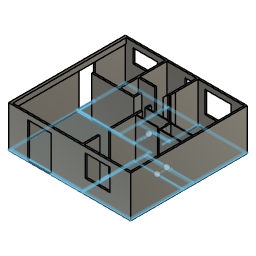
main (Autodesk Fusion 360 design; units mm, degrees)
Autodesk Fusion 360 part; units mm, degrees
note: some values were not read from the file. Set by a fixed rule: which sketch regions a step uses.
sketch "Sketch1" plane through (0, 0, 0) normal (0, 0, 1) x (1, 0, 0)
  line L0 (-340.048, 12.5122) -> (96.952, 12.5122)
  line L1 (96.952, 12.5122) -> (96.952, -391.4878)
  line L2 (96.952, -391.4878) -> (-340.048, -391.4878)
  line L3 (-340.048, -391.4878) -> (-340.048, 12.5122)
  line L4 (-350.048, 22.5122) -> (106.952, 22.5122)
  line L5 (106.952, 22.5122) -> (106.952, -401.4878)
  line L6 (106.952, -401.4878) -> (-350.048, -401.4878)
  line L7 (-350.048, -401.4878) -> (-350.048, 22.5122)
  line L8 (96.952, -391.4878) -> (106.952, -391.4878)
  line L9 (106.952, -391.4878) -> (392.952, -391.4878)
  line L10 (392.952, -391.4878) -> (392.952, -75.4878)
  line L11 (392.952, -75.4878) -> (106.952, -75.4878)
  line L12 (106.952, -75.4878) -> (106.952, -391.4878)
  line L13 (106.952, -401.4878) -> (402.952, -401.4878)
  line L14 (402.952, -401.4878) -> (402.952, -75.4878)
  line L15 (-340.048, 12.5122) -> (-340.048, 22.5122)
  line L16 (96.952, 12.5122) -> (96.952, 22.5122)
  line L17 (-340.048, 22.5122) -> (-93.048, 22.5122)
  line L18 (-93.048, 22.5122) -> (-93.048, 308.5122)
  line L19 (-93.048, 308.5122) -> (-340.048, 308.5122)
  line L20 (-340.048, 308.5122) -> (-340.048, 22.5122)
  line L21 (-350.048, 22.5122) -> (-83.048, 22.5122)
  line L22 (-83.048, 22.5122) -> (-83.048, 318.5122)
  line L23 (-83.048, 318.5122) -> (-350.048, 318.5122)
  line L24 (-350.048, 318.5122) -> (-350.048, 22.5122)
  line L25 (-93.048, 308.5122) -> (-83.048, 308.5122)
  line L26 (-83.048, 308.5122) -> (98.952, 308.5122)
  line L27 (98.952, 308.5122) -> (98.952, 141.5122)
  line L28 (98.952, 141.5122) -> (-83.048, 141.5122)
  line L29 (-83.048, 141.5122) -> (-83.048, 308.5122)
  line L30 (-83.048, 318.5122) -> (108.952, 318.5122)
  line L31 (108.952, 318.5122) -> (108.952, 131.5122)
  line L32 (-83.048, 131.5122) -> (108.952, 131.5122)
  line L33 (98.952, 308.5122) -> (108.952, 308.5122)
  line L34 (108.952, 308.5122) -> (392.952, 308.5122)
  line L35 (392.952, 308.5122) -> (392.952, -7.4878)
  line L36 (392.952, -7.4878) -> (106.952, -7.4878)
  line L37 (108.952, 318.5122) -> (402.952, 318.5122)
  line L38 (402.952, 318.5122) -> (402.952, -75.4878)
  line L39 (392.952, -75.4878) -> (402.952, -75.4878)
  line L40 (106.952, -7.4878) -> (232.2735, -7.4878)
  line L41 (249.952, -75.4878) -> (106.952, -75.4878)
  line L42 (106.952, -75.4878) -> (106.952, -7.4878)
  line L43 (240, -7.4878) -> (392.952, -7.4878)
  line L44 (392.952, -7.4878) -> (392.952, -75.4878)
  line L45 (392.952, -75.4878) -> (240, -75.4878)
  line L46 (106.952, -2.4878) -> (256.952, -2.4878)
  line L47 (256.952, -2.4878) -> (256.952, -20)
  line L48 (256.952, -20) -> (106.952, -20)
  line L49 (106.952, -20) -> (106.952, -2.4878)
  line L50 (392.952, -80.4878) -> (242.952, -80.4878)
  line L51 (242.952, -80.4878) -> (242.952, -20)
  line L52 (242.952, -20) -> (392.952, -20)
  line L53 (392.952, -20) -> (392.952, -80.4878)
  line L54 (106.952, -75.4878) -> (96.952, -75.4878)
  line L55 (96.952, -75.4878) -> (96.952, -230.4878)
  line L56 (96.952, -230.4878) -> (106.952, -230.4878)
  line L57 (106.952, -230.4878) -> (106.952, -75.4878)
  line L58 (96.952, -391.4878) -> (106.952, -391.4878)
  line L59 (106.952, -391.4878) -> (106.952, -295.4878)
  line L60 (106.952, -295.4878) -> (96.952, -295.4878)
  line L61 (96.952, -295.4878) -> (96.952, -391.4878)
  line L62 (-87.7265, -391.4878) -> (79.2735, -391.4878)
  line L63 (79.2735, -391.4878) -> (79.2735, -401.4878)
  line L64 (79.2735, -401.4878) -> (-87.7265, -401.4878)
  line L65 (-87.7265, -401.4878) -> (-87.7265, -391.4878)
  line L66 (-340.048, -391.4878) -> (-232.048, -391.4878)
  line L67 (-232.048, -391.4878) -> (-232.048, -401.4878)
  line L68 (-232.048, -401.4878) -> (-340.048, -401.4878)
  line L69 (-340.048, -401.4878) -> (-340.048, -391.4878)
  line L70 (-251.548, 22.5122) -> (8.452, 22.5122)
  line L71 (8.452, 22.5122) -> (8.452, 12.5122)
  line L72 (8.452, 12.5122) -> (-251.548, 12.5122)
  line L73 (-251.548, 12.5122) -> (-251.548, 22.5122)
  line L74 (-350.048, 22.5122) -> (-340.048, 22.5122)
  line L75 (-340.048, 22.5122) -> (-340.048, 122.5122)
  line L76 (-340.048, 122.5122) -> (-350.048, 122.5122)
  line L77 (-350.048, 122.5122) -> (-350.048, 22.5122)
  line L78 (8.452, 22.5122) -> (-1.548, 22.5122)
  line L79 (-1.548, 22.5122) -> (-1.548, 131.5122)
  line L80 (-1.548, 131.5122) -> (8.452, 131.5122)
  line L81 (8.452, 131.5122) -> (8.452, 22.5122)
  line L82 (-1.548, 131.5122) -> (8.452, 131.5122)
  line L83 (8.452, 131.5122) -> (8.452, 77.0122)
  line L84 (-1.548, 114.5) -> (-1.548, 131.5122)
  line L85 (-1.548, 61.5122) -> (8.452, 61.5122)
  line L86 (98.952, 141.5122) -> (99.322, 141.5122)
  line L87 (99.322, 141.5122) -> (99.322, 102.5122)
  line L88 (99.322, 102.5122) -> (98.952, 102.5122)
  line L89 (98.952, 102.5122) -> (98.952, 141.5122)
  line L90 (18.952, 141.5122) -> (98.952, 141.5122)
  line L91 (98.952, 141.5122) -> (98.952, 131.5122)
  line L92 (98.952, 131.5122) -> (18.952, 131.5122)
  line L93 (18.952, 131.5122) -> (18.952, 141.5122)
  dimension "d1" = 437
  dimension "d2" = 404
  dimension "d3" = 10
  dimension "d4" = 10
  dimension "d5" = 10
  dimension "d6" = 10
  dimension "d7" = 286
  dimension "d9" = 10
  dimension "d10" = 247
  dimension "d11" = 286
  dimension "d12" = 10
  dimension "d13" = 10
  dimension "d14" = 182
  dimension "d15" = 167
  dimension "d16" = 10
  dimension "d17" = 10
  dimension "d19" = 316
  dimension "d20" = 10
  dimension "d21" = 10
  dimension "d22" = 10
  dimension "d23" = 150
  dimension "d24" = 150
  dimension "d25" = 5
  dimension "d26" = 5
  dimension "d27" = 155
  dimension "d28" = 96
  dimension "d29" = 167
  dimension "d30" = 108
  dimension "d31" = 260
  dimension "d32" = 88.5
  dimension "d33" = 88.5
  dimension "d34" = 100
  dimension "d35" = 10
  dimension "d36" = 70
  dimension "d37" = 80
  dimension "d38" = 80
  dimension "d52" = 316
  constraint horizontal L0
  constraint vertical L1
  constraint horizontal L2
  constraint vertical L3
  constraint horizontal L4
  constraint vertical L5
  constraint horizontal L6
  constraint vertical L7
  constraint coincident L5 L8.end
  constraint perpendicular L5 L8
  constraint horizontal L9
  constraint vertical L10
  constraint horizontal L11
  constraint vertical L12
  constraint perpendicular L5 L13
  constraint perpendicular L13 L14
  constraint coincident L4 L15.end
  constraint perpendicular L4 L15
  constraint coincident L4 L16.end
  constraint perpendicular L4 L16
  constraint horizontal L17
  constraint vertical L18
  constraint horizontal L19
  constraint vertical L20
  constraint horizontal L21
  constraint vertical L22
  constraint horizontal L23
  constraint vertical L24
  constraint coincident L22 L25.end
  constraint perpendicular L22 L25
  constraint horizontal L26
  constraint vertical L27
  constraint horizontal L28
  constraint vertical L29
  constraint perpendicular L22 L30
  constraint perpendicular L30 L31
  constraint coincident L22 L32.start
  constraint perpendicular L22 L32
  constraint coincident L31 L33.end
  constraint perpendicular L31 L33
  constraint horizontal L34
  constraint vertical L35
  constraint horizontal L36
  constraint perpendicular L31 L37
  constraint perpendicular L37 L38
  constraint perpendicular L10 L39
  constraint coincident L14.end L39
  constraint coincident L5 L36.end
  constraint horizontal L40
  constraint horizontal L41
  constraint vertical L42
  constraint midpoint L11 L41.start
  constraint horizontal L43
  constraint vertical L44
  constraint horizontal L45
  constraint coincident L36 L43.start
  constraint horizontal L46
  constraint vertical L47
  constraint horizontal L48
  constraint vertical L49
  constraint coincident L5 L46.start
  constraint horizontal L50
  constraint vertical L51
  constraint horizontal L52
  constraint vertical L53
  constraint coincident L48 L51.end
  constraint coincident L10 L50.start
  constraint horizontal L54
  constraint vertical L55
  constraint horizontal L56
  constraint vertical L57
  constraint coincident L1 L55.end
  constraint horizontal L58
  constraint vertical L59
  constraint horizontal L60
  constraint vertical L61
  constraint coincident L5 L59.end
  constraint horizontal L62
  constraint vertical L63
  constraint horizontal L64
  constraint vertical L65
  constraint coincident L6 L63.end
  constraint coincident L2 L62.start
  constraint horizontal L66
  constraint vertical L67
  constraint horizontal L68
  constraint vertical L69
  constraint coincident L6 L67.end
  constraint horizontal L70
  constraint vertical L71
  constraint horizontal L72
  constraint vertical L73
  constraint coincident L0 L71.end
  constraint coincident L17 L70.start
  constraint horizontal L74
  constraint vertical L75
  constraint horizontal L76
  constraint vertical L77
  constraint coincident L20 L75.end
  constraint horizontal L78
  constraint vertical L79
  constraint horizontal L80
  constraint vertical L81
  constraint coincident L32 L79.end
  constraint horizontal L82
  constraint vertical L83
  constraint vertical L84
  constraint midpoint L81 L83.end
  constraint coincident L79 L85.start
  constraint coincident L81 L85.end
  constraint perpendicular L81 L85
  constraint horizontal L86
  constraint vertical L87
  constraint horizontal L88
  constraint vertical L89
  constraint horizontal L90
  constraint vertical L91
  constraint horizontal L92
  constraint vertical L93
  constraint coincident L32 L91.end
  constraint coincident L89 L91.end
  constraint coincident L28 L90.start
  measures "d1" distance of L1.end L2.end
  measures "d2" distance of L0.start L2.end
  measures "d3" distance of L0 L4
  measures "d4" distance of L3 L7
  measures "d5" distance of L1 L5
  measures "d6" distance of L2 L6
  measures "d7" distance of L8.end L9.end
  measures "d9" distance of L10 L14
  measures "d10" distance of L18.end L19.end
  measures "d11" distance of L17.end L18.end
  measures "d12" distance of L19 L23
  measures "d13" distance of L18 L22
  measures "d14" distance of L25.end L26.end
  measures "d15" distance of L26.end L27.end
  measures "d16" distance of L27 L31
  measures "d17" distance of L28 L32
  measures "d19" distance of L34.end L35.end
  measures "d20" distance of L35 L38
  measures "d21" distance of L1 L12
  measures "d22" distance of L34 L37
  measures "d23" distance of L46.start L46.end
  measures "d24" distance of L50.start L50.end
  measures "d25" distance of L36 L46
  measures "d26" distance of L11 L50
  measures "d27" distance of L54 L56
  measures "d28" distance of L58 L60
  measures "d29" distance of L63 L65
  measures "d30" distance of L67 L69
  measures "d31" distance of L71 L73
  measures "d32" distance of L15 L73
  measures "d33" distance of L16 L71
  measures "d34" distance of L74 L76
  measures "d35" distance of L79 L81
  measures "d36" distance of L32 L85
  measures "d37" distance of L4 L88
  measures "d38" distance of L27 L93
  measures "d52" distance of L9 L41
extrude "Extrude1" add sketch "Sketch1" along normal blind 82 contours L3 L4 L6 L7 L15 L21 L69 L74 | L0 L4 L17 L21 L70 L71 L72 L73 L78 | L2 L6 L66 L67 L68 L69 | L19 L20 L22 L23 L24 L25 L76 | L1 L4 L5 L16 L42 L49 L54 | L4 L70 L78 L79 L81 L85 | L4 L18 L21 L22 L25 L29 L70 | L2 L6 L62 L63 L64 L65 | L1 L5 L12 L54 L55 L56 L57 | L2 L5 L6 L8 L58 L63 | L5 L11 L41 L42 L45 L48 L51 | L22 L28 L32 L80 L82 L93 | L22 L26 L30 L31 L33 | L1 L5 L8 L12 L58 L59 L60 L61 | L5 L36 L40 L42 L43 L47 L48 L49 L52 | L5 L36 L40 L43 L46 L47 L49 | L27 L31 L32 L33 L86 L87 | L5 L9 L10 L13 L14 L39 L53 | L31 L34 L35 L37 L38 L39 L44 L53 | L11 L41 L44 L45 L48 L51 L52 L53 | L10 L11 L41 L45 L50 L51 L53 | L32 L86 L87 L89 L91 | L36 L43 L44 L47 L52 | L32 L87 L88 L89 makes body 1 at (-350.048, -260.1544, 27.3333) makes body 2 at (-99.048, 318.5122, 27.3333)
extrude "Extrude2" add sketch "Sketch1" against normal blind 5 separate body makes body 3
sketch "Sketch3" plane through (0, 0, 82) normal (0, 0, 1) x (-1, 0, 0)
  line L0 (83.048, -22.5122) -> (83.048, -131.5122)
  line L1 (-99.322, -131.5122) -> (-108.952, -131.5122)
  line L2 (-18.952, -131.5122) -> (-18.952, -141.5122)
  line L3 (-18.952, -141.5122) -> (83.048, -141.5122)
  line L4 (83.048, -141.5122) -> (83.048, -308.5122)
  line L5 (83.048, -308.5122) -> (-98.952, -308.5122)
  line L6 (-98.952, -308.5122) -> (-98.952, -102.5122)
  line L7 (-98.952, -102.5122) -> (-99.322, -102.5122)
  line L8 (-99.322, -102.5122) -> (-99.322, -131.5122)
  line L9 (-108.952, -308.5122) -> (-392.952, -308.5122)
  line L10 (-392.952, -308.5122) -> (-392.952, 7.4878)
  line L11 (-392.952, 7.4878) -> (-256.952, 7.4878)
  line L12 (-256.952, 7.4878) -> (-256.952, 2.4878)
  line L13 (-256.952, 2.4878) -> (-106.952, 2.4878)
  line L14 (-106.952, 2.4878) -> (-106.952, -22.5122)
  line L15 (-106.952, -22.5122) -> (-96.952, -22.5122)
  line L16 (-96.952, -22.5122) -> (-96.952, 230.4878)
  line L17 (-96.952, 230.4878) -> (-106.952, 230.4878)
  line L18 (-106.952, 230.4878) -> (-106.952, 75.4878)
  line L19 (-106.952, 75.4878) -> (-242.952, 75.4878)
  line L20 (-242.952, 75.4878) -> (-242.952, 80.4878)
  line L21 (-242.952, 80.4878) -> (-392.952, 80.4878)
  line L22 (-392.952, 80.4878) -> (-392.952, 391.4878)
  line L23 (-392.952, 391.4878) -> (-106.952, 391.4878)
  line L24 (-106.952, 391.4878) -> (-106.952, 295.4878)
  line L25 (-106.952, 295.4878) -> (-96.952, 295.4878)
  line L26 (-96.952, 295.4878) -> (-96.952, 391.4878)
  line L27 (-96.952, 391.4878) -> (87.7265, 391.4878)
  line L28 (87.7265, 391.4878) -> (87.7265, 401.4878)
  line L29 (87.7265, 401.4878) -> (-402.952, 401.4878)
  line L30 (-402.952, 401.4878) -> (-402.952, -318.5122)
  line L31 (-402.952, -318.5122) -> (350.048, -318.5122)
  line L32 (350.048, -318.5122) -> (350.048, -122.5122)
  line L33 (350.048, -122.5122) -> (340.048, -122.5122)
  line L34 (340.048, -122.5122) -> (340.048, -308.5122)
  line L35 (340.048, -308.5122) -> (93.048, -308.5122)
  line L36 (93.048, -308.5122) -> (93.048, -22.5122)
  line L37 (93.048, -22.5122) -> (251.548, -22.5122)
  line L38 (251.548, -22.5122) -> (251.548, -12.5122)
  line L39 (251.548, -12.5122) -> (-8.452, -12.5122)
  line L40 (-8.452, -12.5122) -> (-8.452, -61.5122)
  line L41 (-8.452, -61.5122) -> (1.548, -61.5122)
  line L42 (1.548, -61.5122) -> (1.548, -22.5122)
  line L43 (1.548, -22.5122) -> (83.048, -22.5122)
  line L44 (-392.952, 391.4878) -> (-274.952, 391.4878)
  line L45 (-274.952, 391.4878) -> (-274.952, 401.4878)
  line L46 (-274.952, 401.4878) -> (-392.952, 401.4878)
  line L47 (-392.952, 401.4878) -> (-392.952, 391.4878)
  line L48 (-106.952, 391.4878) -> (-122.952, 391.4878)
  line L49 (-122.952, 391.4878) -> (-122.952, 401.4878)
  line L50 (-122.952, 401.4878) -> (-106.952, 401.4878)
  line L51 (-106.952, 401.4878) -> (-106.952, 391.4878)
  line L52 (-392.952, -308.5122) -> (-312.952, -308.5122)
  line L53 (-312.952, -308.5122) -> (-312.952, -318.5122)
  line L54 (-312.952, -318.5122) -> (-392.952, -318.5122)
  line L55 (-392.952, -318.5122) -> (-392.952, -308.5122)
  line L56 (-99.322, -131.5122) -> (-151.322, -131.5122)
  line L57 (-151.322, -131.5122) -> (-151.322, -318.5122)
  line L58 (-151.322, -318.5122) -> (-99.322, -318.5122)
  line L59 (-99.322, -318.5122) -> (-99.322, -131.5122)
  line L60 (-108.952, -131.5122) -> (-108.952, -308.5122)
  line L61 (-99.322, -102.5122) -> (-108.952, -102.5122)
  line L62 (-108.952, -102.5122) -> (-108.952, -131.5122)
  line L63 (-108.952, -131.5122) -> (-99.322, -131.5122)
  line L64 (-99.322, -131.5122) -> (-99.322, -102.5122)
  line L65 (83.048, -131.5122) -> (-18.952, -131.5122)
  dimension "d43" = 118
  dimension "d44" = 80
  dimension "d45" = 52
  dimension "d46" = 152
  constraint horizontal L44
  constraint vertical L45
  constraint horizontal L46
  constraint vertical L47
  constraint coincident L29 L45.end
  constraint coincident L22.end L23.start
  constraint horizontal L48
  constraint vertical L49
  constraint horizontal L50
  constraint vertical L51
  constraint coincident L29 L49.end
  constraint coincident L23.end L24.start
  constraint horizontal L52
  constraint vertical L53
  constraint horizontal L54
  constraint vertical L55
  constraint coincident L31 L53.end
  constraint coincident L9.end L10.start
  constraint horizontal L56
  constraint vertical L57
  constraint horizontal L58
  constraint vertical L59
  constraint coincident L31 L57.end
  constraint coincident L1.start L8.end
  constraint horizontal L61
  constraint vertical L62
  constraint horizontal L63
  constraint vertical L64
  constraint coincident L1.end L60.start
  constraint coincident L7.end L8.start
  measures "d43" distance of L45 L47
  measures "d44" distance of L53 L55
  measures "d45" distance of L57.end L58.end
  measures "d46" distance of L45 L49
extrude "Extrude3" add sketch "Sketch3" 1 faces at (-346.7146, -256.8211, 82) along normal blind 135 contours L0 L2 L3 L4 L5 L6 L7 L8 L31 L32 L33 L34 L35 L36 L37 L38 L39 L40 L41 L42 L43 L59 L64 L65 | L1 L9 L31 L56 L57 L58 L59 L60 L63 | L9 L31 L52 L53 L54 L55 | L10 L11 L12 L13 L14 L15 L16 L17 L18 L19 L20 L21 L22 L29 L30 L31 L47 L55 | L23 L29 L44 L45 L46 L47 | L23 L29 L48 L49 L50 L51 | L24 L25 L26 L27 L28 L29 L51 on bodies 1 bodies 1 2 3
sketch "Sketch6" plane through (0, 0, 0) normal (0, 0, 1) x (1, 0, 0)
  line L0 (109, 169) -> (99, 169)
  line L1 (99, 169) -> (99, 140)
  line L2 (99, 140) -> (109, 140)
  line L3 (109, 140) -> (109, 169)
  constraint horizontal L0
  constraint vertical L1
  constraint horizontal L2
  constraint vertical L3
extrude "Extrude4" add sketch "Sketch6" along normal blind 217 bodies 2 3
sketch "Sketch7" plane through (0, 0, 217) normal (0, 0, 1) x (-1, 0, 0)
  line L0 (-98.952, -102.5122) -> (-99.322, -102.5122)
  line L1 (-109, -140) -> (-109, -169)
  line L2 (-109, -169) -> (-108.952, -169)
  line L3 (-108.952, -169) -> (-108.952, -308.5122)
  line L4 (-108.952, -308.5122) -> (-151.322, -308.5122)
  line L5 (-151.322, -308.5122) -> (-151.322, -318.5122)
  line L6 (-151.322, -318.5122) -> (350.048, -318.5122)
  line L7 (350.048, -318.5122) -> (350.048, -122.5122)
  line L8 (350.048, -122.5122) -> (340.048, -122.5122)
  line L9 (340.048, -122.5122) -> (340.048, -308.5122)
  line L10 (340.048, -308.5122) -> (93.048, -308.5122)
  line L11 (93.048, -308.5122) -> (93.048, -22.5122)
  line L12 (93.048, -22.5122) -> (251.548, -22.5122)
  line L13 (251.548, -22.5122) -> (251.548, -12.5122)
  line L14 (251.548, -12.5122) -> (-8.452, -12.5122)
  line L15 (-8.452, -12.5122) -> (-8.452, -61.5122)
  line L16 (-8.452, -61.5122) -> (1.548, -61.5122)
  line L17 (1.548, -61.5122) -> (1.548, -22.5122)
  line L18 (1.548, -22.5122) -> (83.048, -22.5122)
  line L19 (83.048, -22.5122) -> (83.048, -131.5122)
  line L20 (83.048, -131.5122) -> (-18.952, -131.5122)
  line L21 (-18.952, -131.5122) -> (-18.952, -141.5122)
  line L22 (-18.952, -141.5122) -> (83.048, -141.5122)
  line L23 (83.048, -141.5122) -> (83.048, -308.5122)
  line L24 (83.048, -308.5122) -> (-98.952, -308.5122)
  line L25 (-98.952, -308.5122) -> (-98.952, -102.5122)
  line L26 (-98.952, -308.5122) -> (-28.952, -308.5122)
  line L27 (-28.952, -308.5122) -> (-28.952, -318.5122)
  line L28 (-28.952, -318.5122) -> (-98.952, -318.5122)
  line L29 (-98.952, -318.5122) -> (-98.952, -308.5122)
  line L30 (291.548, -318.5122) -> (141.548, -318.5122)
  line L31 (141.548, -318.5122) -> (141.548, -308.5122)
  line L32 (141.548, -308.5122) -> (291.548, -308.5122)
  line L33 (291.548, -308.5122) -> (291.548, -318.5122)
  line L34 (340.048, -308.5122) -> (340.048, -22.5122)
  line L35 (93.048, -22.5122) -> (93.048, -308.5122)
  line L36 (-99.322, -102.5122) -> (-99.322, -131.5122)
  line L37 (-99.322, -131.5122) -> (-108.952, -131.5122)
  line L38 (-108.952, -131.5122) -> (-108.952, -140)
  line L39 (-108.952, -140) -> (-109, -140)
  dimension "d55" = 70
  dimension "d56" = 150
  dimension "d57" = 48.5
  dimension "d58" = 48.5
  constraint horizontal L26
  constraint vertical L27
  constraint horizontal L28
  constraint vertical L29
  constraint coincident L6 L27.end
  constraint coincident L24.end L25.start
  constraint horizontal L30
  constraint vertical L31
  constraint horizontal L32
  constraint vertical L33
  constraint coincident L10 L31.end
  constraint coincident L6 L30.start
  measures "d55" distance of L27 L29
  measures "d56" distance of L31 L33
  measures "d57" distance of L33 L34
  measures "d58" distance of L31 L35
extrude "Extrude5" cut sketch "Sketch7" against normal blind 75 contours L6 L24 L26 L27 L28 L29 | L6 L10 L30 L31 L32 L33 bodies 2
extrude "Extrude6" cut 1 faces at (-191.548, 315.1789, 142) along direction (0, 0, -1) blind 10 on bodies 2 bodies 2
sketch "Sketch8" plane through (0, 0, 217) normal (0, 0, 1) x (-1, 0, 0)
  line L0 (340.048, 391.4878) -> (340.048, -22.5122)
  line L1 (340.048, -22.5122) -> (350.048, -22.5122)
  line L2 (350.048, -22.5122) -> (350.048, 401.4878)
  line L3 (350.048, 401.4878) -> (232.048, 401.4878)
  line L4 (232.048, 401.4878) -> (232.048, 391.4878)
  line L5 (232.048, 391.4878) -> (340.048, 391.4878)
  line L6 (350.048, 401.4878) -> (334.4798, 401.4878)
  line L7 (334.4798, 401.4878) -> (334.4798, -318.5122)
  line L8 (334.4798, -318.5122) -> (350.048, -318.5122)
  line L9 (350.048, -318.5122) -> (350.048, 401.4878)
  line L10 (350.048, -318.5122) -> (-402.952, -318.5122)
  line L11 (-402.952, -318.5122) -> (-402.952, -308.5122)
  line L12 (-402.952, -308.5122) -> (350.048, -308.5122)
  line L13 (350.048, -308.5122) -> (350.048, -318.5122)
  line L14 (83.048, -318.5122) -> (350.048, -318.5122)
  line L15 (93.048, -308.5122) -> (340.048, -308.5122)
  line L16 (-402.952, -308.5122) -> (-392.952, -308.5122)
  line L17 (-392.952, -308.5122) -> (-392.952, 401.4878)
  line L18 (-392.952, 401.4878) -> (-402.952, 401.4878)
  line L19 (-402.952, 401.4878) -> (-402.952, -308.5122)
  line L20 (334.4798, 401.4878) -> (-392.952, 401.4878)
  line L21 (-392.952, 401.4878) -> (-392.952, 391.4878)
  line L22 (-392.952, 391.4878) -> (334.4798, 391.4878)
  line L23 (334.4798, 391.4878) -> (334.4798, 401.4878)
  point P0 (-402.952, -318.5122)
  point P1 (-402.952, 401.4878)
  point P2 (-392.952, 391.4878)
  constraint horizontal L6
  constraint vertical L7
  constraint horizontal L8
  constraint vertical L9
  constraint coincident L2.end L3.start
  constraint horizontal L10
  constraint vertical L11
  constraint horizontal L12
  constraint vertical L13
  constraint collinear L10 L14
  constraint collinear L12 L15
  constraint coincident L11 P0
  constraint horizontal L16
  constraint vertical L17
  constraint horizontal L18
  constraint vertical L19
  constraint coincident L18 P1
  constraint coincident L17 P2
  constraint horizontal L20
  constraint vertical L21
  constraint horizontal L22
  constraint vertical L23
  constraint coincident P2 L21.end
extrude "Extrude8" add sketch "Sketch8" along normal blind 33 contours L0 L1 L2 L3 L5 L6 L7 L9 L23 | L0 L1 L5 L7 L9 L12 L15 | L3 L4 L5 L7 L20 L22 L23 | L4 L17 L20 L21 L22 | L7 L8 L9 L10 L12 L13 L14 L15 | L7 L10 L11 L12 L14 L15 L16 | L12 L16 L17 L18 L19 L21 bodies 1 2
extrude "Extrude9" add 4 faces at (103.6187, -359.4878, 217) (297.6187, -54.4878, 217) (102.4087, 203.0082, 217) (-89.7146, 154.1789, 217) along direction (0, 0, 1) blind 33 on bodies 1 bodies 1
sketch "Sketch9" plane through (0, 0, 250) normal (0, 0, 1) x (-1, 0, 0)
  line L0 (334.4798, -308.5122) -> (93.048, -308.5122)
  line L1 (93.048, -308.5122) -> (93.048, -22.5122)
  line L2 (93.048, -22.5122) -> (251.548, -22.5122)
  line L3 (251.548, -22.5122) -> (251.548, -12.5122)
  line L4 (251.548, -12.5122) -> (-8.452, -12.5122)
  line L5 (-8.452, -12.5122) -> (-8.452, -61.5122)
  line L6 (-8.452, -61.5122) -> (1.548, -61.5122)
  line L7 (1.548, -61.5122) -> (1.548, -22.5122)
  line L8 (1.548, -22.5122) -> (83.048, -22.5122)
  line L9 (83.048, -22.5122) -> (83.048, -131.5122)
  line L10 (83.048, -131.5122) -> (-18.952, -131.5122)
  line L11 (-18.952, -131.5122) -> (-18.952, -141.5122)
  line L12 (-18.952, -141.5122) -> (83.048, -141.5122)
  line L13 (83.048, -141.5122) -> (83.048, -308.5122)
  line L14 (83.048, -308.5122) -> (-98.952, -308.5122)
  line L15 (-98.952, -308.5122) -> (-98.952, -102.5122)
  line L16 (-98.952, -102.5122) -> (-99.322, -102.5122)
  line L17 (-109, -140) -> (-109, -169)
  line L18 (-109, -169) -> (-108.952, -169)
  line L19 (-99.322, -102.5122) -> (-99.322, -131.5122)
  line L20 (-108.952, -308.5122) -> (-392.952, -308.5122)
  line L21 (-392.952, -308.5122) -> (-392.952, 7.4878)
  line L22 (-392.952, 7.4878) -> (-256.952, 7.4878)
  line L23 (-256.952, 7.4878) -> (-256.952, 2.4878)
  line L24 (-256.952, 2.4878) -> (-106.952, 2.4878)
  line L25 (-106.952, 2.4878) -> (-106.952, -22.5122)
  line L26 (-106.952, -22.5122) -> (-96.952, -22.5122)
  line L27 (-96.952, -22.5122) -> (-96.952, 230.4878)
  line L28 (-96.952, 230.4878) -> (-106.952, 230.4878)
  line L29 (-106.952, 230.4878) -> (-106.952, 75.4878)
  line L30 (-106.952, 75.4878) -> (-242.952, 75.4878)
  line L31 (-242.952, 75.4878) -> (-242.952, 80.4878)
  line L32 (-242.952, 80.4878) -> (-392.952, 80.4878)
  line L33 (-392.952, 80.4878) -> (-392.952, 391.4878)
  line L34 (-392.952, 391.4878) -> (-106.952, 391.4878)
  line L35 (-106.952, 391.4878) -> (-106.952, 295.4878)
  line L36 (-106.952, 295.4878) -> (-96.952, 295.4878)
  line L37 (-96.952, 295.4878) -> (-96.952, 391.4878)
  line L38 (-96.952, 391.4878) -> (334.4798, 391.4878)
  line L39 (334.4798, 391.4878) -> (334.4798, -308.5122)
  line L40 (350.048, -318.5122) -> (350.048, 401.4878)
  line L41 (350.048, 401.4878) -> (-402.952, 401.4878)
  line L42 (-402.952, 401.4878) -> (-402.952, -318.5122)
  line L43 (-402.952, -318.5122) -> (350.048, -318.5122)
  line L44 (-106.952, 7.4878) -> (-251.952, 7.4878)
  line L45 (-251.952, 7.4878) -> (-251.952, 70.4878)
  line L46 (-251.952, 70.4878) -> (-106.952, 70.4878)
  line L47 (-106.952, 70.4878) -> (-106.952, 7.4878)
  line L48 (-261.952, 12.4878) -> (-392.952, 12.4878)
  line L49 (-392.952, 12.4878) -> (-392.952, 75.4878)
  line L50 (-392.952, 75.4878) -> (-261.952, 75.4878)
  line L51 (-261.952, 75.4878) -> (-261.952, 12.4878)
  line L52 (-106.952, 2.4878) -> (-256.952, 2.4878)
  line L53 (-392.952, 75.4878) -> (-106.952, 75.4878)
  line L54 (-392.952, 7.4878) -> (-106.952, 7.4878)
  line L55 (-392.952, 80.4878) -> (-242.952, 80.4878)
  line L56 (-392.952, -308.5122) -> (-392.952, 7.4878)
  line L57 (-106.952, -22.5122) -> (-106.952, 401.4878)
  line L58 (-99.322, -131.5122) -> (-108.952, -131.5122)
  line L59 (-108.952, -131.5122) -> (-108.952, -140)
  line L60 (-108.952, -140) -> (-109, -140)
  line L61 (-108.952, -169) -> (-108.952, -308.5122)
  dimension "d69" = 5
  dimension "d70" = 5
  dimension "d71" = 5
  dimension "d72" = 5
  dimension "d73" = 5
  dimension "d74" = 5
  constraint horizontal L44
  constraint vertical L45
  constraint horizontal L46
  constraint vertical L47
  constraint horizontal L48
  constraint vertical L49
  constraint horizontal L50
  constraint vertical L51
  constraint collinear L49 L56
  constraint collinear L47 L57
  measures "d69" distance of L44 L52
  measures "d70" distance of L46 L53
  measures "d71" distance of L45 L23.end
  measures "d72" distance of L48 L54
  measures "d73" distance of L50 L55
  measures "d74" distance of L51 L23.end
extrude "Extrude10" cut sketch "Sketch9" against normal blind 250 contours L44 L45 L46 L47 L54 L57 | L48 L49 L50 L51 L53 bodies 1
sketch "Sketch10" plane through (0, 0, 250) normal (0, 0, 1) x (-1, 0, 0)
  line L0 (-106.952, 7.4878) -> (-251.952, 7.4878)
  line L1 (-251.952, 7.4878) -> (-251.952, 70.4878)
  line L2 (-251.952, 70.4878) -> (-106.952, 70.4878)
  line L3 (-106.952, 70.4878) -> (-106.952, 7.4878)
  line L4 (-261.952, 12.4878) -> (-392.952, 12.4878)
  line L5 (-392.952, 12.4878) -> (-392.952, 75.4878)
  line L6 (-392.952, 75.4878) -> (-261.952, 75.4878)
  line L7 (-261.952, 75.4878) -> (-261.952, 12.4878)
  line L8 (334.4798, -308.5122) -> (93.048, -308.5122)
  line L9 (93.048, -308.5122) -> (93.048, -22.5122)
  line L10 (93.048, -22.5122) -> (251.548, -22.5122)
  line L11 (251.548, -22.5122) -> (251.548, -12.5122)
  line L12 (251.548, -12.5122) -> (-8.452, -12.5122)
  line L13 (-8.452, -12.5122) -> (-8.452, -61.5122)
  line L14 (-8.452, -61.5122) -> (1.548, -61.5122)
  line L15 (1.548, -61.5122) -> (1.548, -22.5122)
  line L16 (1.548, -22.5122) -> (83.048, -22.5122)
  line L17 (83.048, -22.5122) -> (83.048, -131.5122)
  line L18 (83.048, -131.5122) -> (-18.952, -131.5122)
  line L19 (-18.952, -131.5122) -> (-18.952, -141.5122)
  line L20 (-18.952, -141.5122) -> (83.048, -141.5122)
  line L21 (83.048, -141.5122) -> (83.048, -308.5122)
  line L22 (83.048, -308.5122) -> (-98.952, -308.5122)
  line L23 (-98.952, -308.5122) -> (-98.952, -102.5122)
  line L24 (-98.952, -102.5122) -> (-99.322, -102.5122)
  line L25 (-109, -140) -> (-109, -169)
  line L26 (-109, -169) -> (-108.952, -169)
  line L27 (-99.322, -102.5122) -> (-99.322, -131.5122)
  line L28 (-108.952, -308.5122) -> (-392.952, -308.5122)
  line L29 (-392.952, -308.5122) -> (-392.952, 7.4878)
  line L30 (-392.952, 7.4878) -> (-256.952, 7.4878)
  line L31 (-256.952, 7.4878) -> (-256.952, 2.4878)
  line L32 (-256.952, 2.4878) -> (-106.952, 2.4878)
  line L33 (-106.952, 2.4878) -> (-106.952, -22.5122)
  line L34 (-106.952, -22.5122) -> (-96.952, -22.5122)
  line L35 (-96.952, -22.5122) -> (-96.952, 230.4878)
  line L36 (-96.952, 230.4878) -> (-106.952, 230.4878)
  line L37 (-106.952, 230.4878) -> (-106.952, 75.4878)
  line L38 (-106.952, 75.4878) -> (-242.952, 75.4878)
  line L39 (-242.952, 75.4878) -> (-242.952, 80.4878)
  line L40 (-242.952, 80.4878) -> (-392.952, 80.4878)
  line L41 (-392.952, 80.4878) -> (-392.952, 391.4878)
  line L42 (-392.952, 391.4878) -> (-106.952, 391.4878)
  line L43 (-106.952, 391.4878) -> (-106.952, 295.4878)
  line L44 (-106.952, 295.4878) -> (-96.952, 295.4878)
  line L45 (-96.952, 295.4878) -> (-96.952, 391.4878)
  line L46 (-96.952, 391.4878) -> (334.4798, 391.4878)
  line L47 (334.4798, 391.4878) -> (334.4798, -308.5122)
  line L48 (350.048, -318.5122) -> (350.048, 401.4878)
  line L49 (350.048, 401.4878) -> (-402.952, 401.4878)
  line L50 (-402.952, 401.4878) -> (-402.952, -318.5122)
  line L51 (-402.952, -318.5122) -> (350.048, -318.5122)
  line L52 (-242.952, 80.4878) -> (-256.952, 80.4878)
  line L53 (-256.952, 80.4878) -> (-256.952, 38)
  line L54 (-256.952, 38) -> (-242.952, 38)
  line L55 (-242.952, 38) -> (-242.952, 80.4878)
  line L56 (-99.322, -131.5122) -> (-108.952, -131.5122)
  line L57 (-108.952, -131.5122) -> (-108.952, -140)
  line L58 (-108.952, -140) -> (-109, -140)
  line L59 (-108.952, -169) -> (-108.952, -308.5122)
  dimension "d77" = 5
  constraint horizontal L52
  constraint vertical L53
  constraint horizontal L54
  constraint vertical L55
  constraint coincident L39.end L40.start
  measures "d77" distance of L7 L53
extrude "Extrude11" cut sketch "Sketch10" against normal blind 250 contours L1 L2 L39 L40 L52 L53 L54 L55 | L1 L2 L54 L55 bodies 1
sketch "Sketch11" plane through (0, 0, 250) normal (0, 0, 1) x (-1, 0, 0)
  line L0 (350.048, -318.5122) -> (350.048, 401.4878)
  line L1 (350.048, 401.4878) -> (-402.952, 401.4878)
  line L2 (-402.952, 401.4878) -> (-402.952, -318.5122)
  line L3 (-402.952, -318.5122) -> (350.048, -318.5122)
  line L4 (-106.952, 75.4878) -> (-242.952, 75.4878)
  line L5 (-256.952, 38) -> (-256.952, 80.4878)
  line L6 (-256.952, 80.4878) -> (-392.952, 80.4878)
  line L7 (-392.952, 80.4878) -> (-392.952, 391.4878)
  line L8 (-392.952, 391.4878) -> (-106.952, 391.4878)
  line L9 (-106.952, 391.4878) -> (-106.952, 295.4878)
  line L10 (-106.952, 295.4878) -> (-96.952, 295.4878)
  line L11 (-96.952, 295.4878) -> (-96.952, 391.4878)
  line L12 (-96.952, 391.4878) -> (334.4798, 391.4878)
  line L13 (334.4798, 391.4878) -> (334.4798, -308.5122)
  line L14 (334.4798, -308.5122) -> (93.048, -308.5122)
  line L15 (93.048, -308.5122) -> (93.048, -22.5122)
  line L16 (93.048, -22.5122) -> (251.548, -22.5122)
  line L17 (251.548, -22.5122) -> (251.548, -12.5122)
  line L18 (251.548, -12.5122) -> (-8.452, -12.5122)
  line L19 (-8.452, -12.5122) -> (-8.452, -61.5122)
  line L20 (-8.452, -61.5122) -> (1.548, -61.5122)
  line L21 (1.548, -61.5122) -> (1.548, -22.5122)
  line L22 (1.548, -22.5122) -> (83.048, -22.5122)
  line L23 (83.048, -22.5122) -> (83.048, -131.5122)
  line L24 (83.048, -131.5122) -> (-18.952, -131.5122)
  line L25 (-18.952, -131.5122) -> (-18.952, -141.5122)
  line L26 (-18.952, -141.5122) -> (83.048, -141.5122)
  line L27 (83.048, -141.5122) -> (83.048, -308.5122)
  line L28 (83.048, -308.5122) -> (-98.952, -308.5122)
  line L29 (-98.952, -308.5122) -> (-98.952, -102.5122)
  line L30 (-98.952, -102.5122) -> (-99.322, -102.5122)
  line L31 (-109, -140) -> (-109, -169)
  line L32 (-109, -169) -> (-108.952, -169)
  line L33 (-99.322, -102.5122) -> (-99.322, -131.5122)
  line L34 (-108.952, -308.5122) -> (-392.952, -308.5122)
  line L35 (-392.952, -308.5122) -> (-392.952, 7.4878)
  line L36 (-392.952, 7.4878) -> (-256.952, 7.4878)
  line L37 (-256.952, 7.4878) -> (-256.952, 2.4878)
  line L38 (-256.952, 2.4878) -> (-106.952, 2.4878)
  line L39 (-106.952, 2.4878) -> (-106.952, -22.5122)
  line L40 (-106.952, -22.5122) -> (-96.952, -22.5122)
  line L41 (-96.952, -22.5122) -> (-96.952, 230.4878)
  line L42 (-96.952, 230.4878) -> (-106.952, 230.4878)
  line L43 (-106.952, 230.4878) -> (-106.952, 75.4878)
  line L44 (-261.952, 12.4878) -> (-392.952, 12.4878)
  line L45 (-392.952, 12.4878) -> (-392.952, 75.4878)
  line L46 (-392.952, 75.4878) -> (-261.952, 75.4878)
  line L47 (-261.952, 75.4878) -> (-261.952, 12.4878)
  line L48 (-106.952, 7.4878) -> (-251.952, 7.4878)
  line L49 (-251.952, 7.4878) -> (-251.952, 38)
  line L50 (-242.952, 70.4878) -> (-106.952, 70.4878)
  line L51 (-106.952, 70.4878) -> (-106.952, 7.4878)
  line L52 (-106.952, 7.4878) -> (-96.952, 7.4878)
  line L53 (-96.952, 7.4878) -> (-96.952, 33)
  line L54 (-96.952, 33) -> (-106.952, 33)
  line L55 (-106.952, 33) -> (-106.952, 7.4878)
  line L56 (-99.322, -131.5122) -> (-108.952, -131.5122)
  line L57 (-108.952, -131.5122) -> (-108.952, -140)
  line L58 (-108.952, -140) -> (-109, -140)
  line L59 (-108.952, -169) -> (-108.952, -308.5122)
  line L60 (-242.952, 75.4878) -> (-242.952, 70.4878)
  line L61 (-251.952, 38) -> (-256.952, 38)
  constraint horizontal L52
  constraint vertical L53
  constraint horizontal L54
  constraint vertical L55
  constraint coincident L41 L53.end
  constraint coincident L48.start L51.end
extrude "Extrude12" cut sketch "Sketch11" against normal blind 250 contours L41 L51 L52 L53 L54 L55 bodies 1
